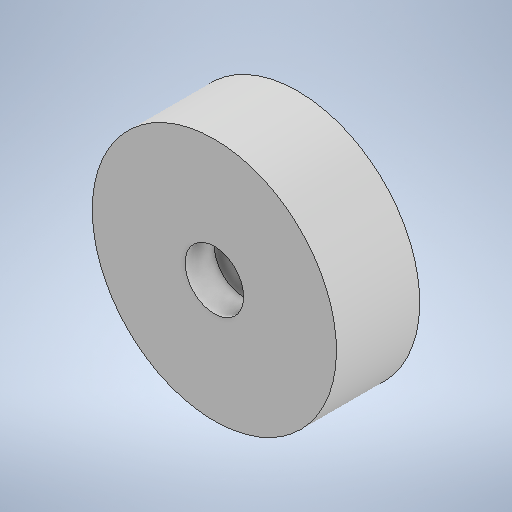
# Autodesk Inventor part: Back Cover seal
Saved by Autodesk Inventor 2026.2 (Build 302298000, 298)
## iProperties
Created: 2026-01-18
Part Number: Back Cover seal
Material: Generic
Document SubType Name: Modeling
Designer: daryu
Density: 1 g/cm^3
Appearance: Default
Author: daryu
Autodesk Inventor part; units mm, degrees
ref_plane "YZ Plane" through (0, 0, 0) normal (1, 0, 0) x (0, 1, 0)
ref_plane "XZ Plane" through (0, 0, 0) normal (0, 1, 0) x (-1, 0, 0)
ref_plane "XY Plane" through (0, 0, 0) normal (0, 0, 1) x (1, 0, 0)
sketch "Sketch1" plane through (0, 0, 0) normal (1, 0, 0) x (0, 1, 0)
  line L0 (-1.7337, 8.6435) -> (-1.7337, 9.8775)
  line L1 (-1.7337, 9.8775) -> (10.7663, 9.8775)
  line L2 (10.7663, 8.6435) -> (10.7663, 9.8775)
  line L3 (-1.7337, 5.6125) -> (10.7663, 5.6125)
  line L4 (-1.7337, 9.8775) -> (-1.7337, 5.6125)
  line L5 (10.7663, 9.8775) -> (10.7663, 5.6125)
  arc A0 (10.7663, 5.6125) -> (-1.7337, 5.6125) centre (4.5163, -3.4255) ccw
  line L6 (4.5163, 9.8775) -> (4.5163, 5.6125)
  point P0 (0, 0)
  point P1 (4.5163, 7.5631)
  constraints: 14 end point, 3 vertical, 2 midpoint, 2 point on circle, 1 centre point, 1 perpendicular, 3 other
revolve "Revolution1" add sketch "Sketch1" angle 360 about axis through (0, 4.5163, 9.8775) along (0, 0, -1) contours L1 L2 L5 A0 L6
sketch "Sketch2" plane through (0, 4.5163, 9.8775) normal (0, 0, 1) x (1, 0, 0)
  circle A0 centre (0, 0) radius 1.5
  point P0 (0, -4.5163)
  dimension "d1" = 3
  constraints: 1 centre point
  measures "d1" diameter of A0
hole "Hole1" at (0, 4.5163, 9.8775) direction (0, 0, -1) diameter 3 depth 1.5
body "Solid1"
